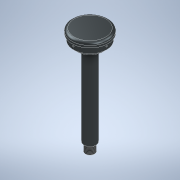
# Autodesk Inventor part: Сапун
Saved by Autodesk Inventor 2021 (Build 250183000, 183)
## iProperties
Created: 2020-12-21
Part Number: Сапун
Material: Чугун, серый
Document SubType Name: Modeling
Designer: Тимоха
Mass: 2294.86 g
Surface Area: 1318.55 cm^2
Volume: 320.96 cm^3
Density: 7.15 g/cm^3
Appearance: Чугун серый
Author: Тимоха
Autodesk Inventor part; units mm, degrees
ref_plane "YZ Plane" through (0, 0, 0) normal (1, 0, 0) x (0, 1, 0)
ref_plane "XZ Plane" through (0, 0, 0) normal (0, 1, 0) x (-1, 0, 0)
ref_plane "XY Plane" through (0, 0, 0) normal (0, 0, 1) x (1, 0, 0)
sketch "Эскиз1" plane through (0, 0, 0) normal (0, 0, 1) x (1, 0, 0)
  line L0 (0, 0) -> (15, 0)
  line L1 (15, 0) -> (15, 30)
  line L2 (15, 30) -> (20, 30)
  line L3 (20, 30) -> (20, 310)
  line L4 (20, 310) -> (45, 310)
  line L5 (45, 310) -> (45, 320)
  line L6 (45, 320) -> (55, 320)
  line L7 (55, 320) -> (55, 340)
  line L8 (55, 340) -> (60, 340)
  line L9 (60, 340) -> (60, 347)
  line L10 (52, 355) -> (0, 355)
  arc A0 (60, 347) -> (52, 355) centre (52, 347) ccw
  line L11 (15, 0) -> (10, 0)
  line L12 (10, 0) -> (10, 35)
  line L13 (10, 35) -> (15, 35)
  line L14 (15, 35) -> (15, 315)
  line L15 (15, 315) -> (40, 315)
  line L16 (40, 315) -> (40, 325)
  line L17 (40, 325) -> (50, 325)
  line L18 (50, 325) -> (50, 343.5)
  line L19 (50, 343.5) -> (55, 343.5)
  line L20 (55, 343.5) -> (55, 346.5)
  line L21 (51, 350.5) -> (0, 350.5)
  arc A1 (55, 346.5) -> (51, 350.5) centre (51, 346.5) ccw
  line L22 (0, 355) -> (0, 350.5)
  point P0 (60, 355)
  dimension "d0" = 15
  dimension "d1" = 30
  dimension "d2" = 5
  dimension "d3" = 280
  dimension "d4" = 25
  dimension "d5" = 10
  dimension "d6" = 10
  dimension "d7" = 20
  dimension "d8" = 5
  dimension "d9" = 15
  dimension "d10" = 8
  dimension "d11" = 5
  dimension "d12" = 35
  dimension "d13" = 25
  dimension "d14" = 10
  dimension "d15" = 10
  dimension "d16" = 18.5
  dimension "d17" = 4
  dimension "d18" = 3
  constraints: 46 end point, 16 perpendicular, 4 point on circle, 4 tangent, 3 horizontal, 3 point on line, 2 centre point, 2 vertical, 1 parallel
  measures "d0" distance of L0.start L0.end
  measures "d1" distance of L0.end L1.end
  measures "d2" distance of L1.end L2.end
  measures "d3" distance of L2.end L3.end
  measures "d4" distance of L3.end L4.end
  measures "d5" distance of L4.end L5.end
  measures "d6" distance of L5.end L6.end
  measures "d7" distance of L6.end L7.end
  measures "d8" distance of L7.end L8.end
  measures "d9" distance of L8.end point (60, 355)
  measures "d10" radius of A0
  measures "d11" distance of L0.end L11.end
  measures "d12" distance of L11.end L12.end
  measures "d13" distance of L14.end L15.end
  measures "d14" distance of L15.end L16.end
  measures "d15" distance of L16.end L17.end
  measures "d16" distance of L17.end L18.end
  measures "d17" radius of A1
  measures "d18" distance of L19.end L20.end
revolve "Вращение1" add sketch "Эскиз1" angle 360 about axis through (0, 355, 0) along (0, -1, 0)
sketch "Эскиз2" plane through (0, 0, 0) normal (1, 0, 0) x (0, 1, 0)
  line L0 (340, 55) -> (340, -55) projected
  line L1 (320, 55) -> (320, -55) projected
  circle A0 centre (330, 0) radius 2.5
  point P0 (0, 0)
  dimension "d20" = 5
  constraints: 1 centre point
  measures "d20" diameter of A0
extrude "Выдавливание1" cut sketch "Эскиз2" against normal through all both and the other way through all
pattern_circular "Круговой массив1" count 4 over 360 about axis through (0, 330, 0) along (0, -1, 0) of "Выдавливание1"
thread "Резьба1" size "M30x3.5" class "6g" standard "ANSI Metric M Profile" full length
chamfer "Фаска1" distance 2 angle 45 1 edges at (-15, 0, 0)
